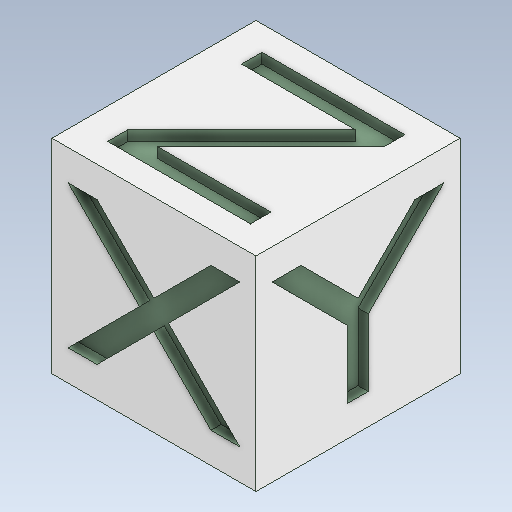
# Autodesk Inventor part: Cubo-0001-002
Saved by Autodesk Inventor 2025.2 (Build 292293000, 293)
## iProperties
Created: 2025-01-15
Part Number: Cubo-0001-002
Material: Borracha
Document SubType Name: Modeling
Designer: Gustavo Sousa
Density: 0.93 g/cm^3
Appearance: Borracha - Verde
Author: Gustavo Sousa
Autodesk Inventor part; units mm, degrees
ref_plane "YZ Plane" through (0, 0, 0) normal (1, 0, 0) x (0, 1, 0)
ref_plane "XZ Plane" through (0, 0, 0) normal (0, 1, 0) x (-1, 0, 0)
ref_plane "XY Plane" through (0, 0, 0) normal (0, 0, 1) x (1, 0, 0)
sketch "Esboço1" plane through (0, 0, 0) normal (0, 0, 1) x (1, 0, 0)
  line L0 (-10, -10) -> (10, -10)
  line L1 (10, -10) -> (10, 10)
  line L2 (10, 10) -> (-10, 10)
  line L3 (-10, 10) -> (-10, -10)
  line L4 (-10, -10) -> (10, 10) construction
  line L5 (10, -10) -> (-10, 10) construction
  point P0 (0, 0)
  dimension "d0" = 20
  dimension "d1" = 20
  constraints: 12 end point, 2 midpoint, 2 parallel, 1 horizontal, 1 perpendicular
  measures "d0" distance of L2.end L1.end
  measures "d1" distance of L1.end L0.end
extrude "Extrusão1" add sketch "Esboço1" along normal mid plane 20
sketch "Esboço4" plane through (0, 0, 10) normal (0, 0, 1) x (1, 0, 0)
  line L0 (-7, -7) -> (7, -7) construction
  line L1 (7, -7) -> (7, 7) construction
  line L2 (7, 7) -> (-7, 7) construction
  line L3 (-7, 7) -> (-7, -7) construction
  line L4 (0, 1.4142) -> (-1.4142, 0)
  line L5 (-1.4142, 0) -> (0, -1.4142)
  line L6 (0, -1.4142) -> (1.4142, 0)
  line L7 (1.4142, 0) -> (0, 1.4142)
  line L8 (0, 1.4142) -> (0, -1.4142) construction
  line L9 (-1.4142, 0) -> (1.4142, 0) construction
  line L10 (0, -1.4142) -> (1.4142, 0)
  line L11 (1.4142, 0) -> (7.0002, -5.586)
  line L12 (5.586, -7.0002) -> (0, -1.4142)
  line L13 (0, -1.4142) -> (-1.4142, 0)
  line L14 (-1.4142, 0) -> (-7.0001, -5.5859)
  line L15 (-5.5859, -7.0001) -> (0, -1.4142)
  line L16 (-1.4142, 0) -> (0, 1.4142)
  line L17 (0, 1.4142) -> (-5.5858, 7)
  line L18 (-7, 5.5858) -> (-1.4142, 0)
  line L19 (1.4142, 0) -> (0, 1.4142)
  line L20 (0, 1.4142) -> (5.5858, 7)
  line L21 (7, 5.5858) -> (1.4142, 0)
  line L22 (-8.4142, 7) -> (-7, 5.5858)
  line L23 (7, 5.5858) -> (8.4142, 7)
  line L24 (8.4142, -7) -> (7, -5.5858)
  line L25 (-7, -5.5858) -> (-8.4142, -7)
  line L26 (-5.5858, -7) -> (-8.4142, -7)
  line L27 (5.5858, -7) -> (7, -7)
  line L28 (7, -7) -> (8.4142, -7)
  line L29 (-5.5858, 7) -> (-8.4142, 7)
  line L30 (5.5858, 7) -> (7, 7)
  line L31 (7, 7) -> (8.4142, 7)
  point P0 (0, 0)
  point P1 (0, 0)
  point P2 (-7, 7)
  point P3 (-7, -7)
  point P4 (6.2929, 7)
  point P5 (7.7071, -7)
  dimension "d62" = 2
  dimension "d63" = 2
  dimension "d64" = 14
  dimension "d65" = 14
  dimension "d68" = 2
  dimension "d69" = 2
  dimension "d70" = 2
  dimension "d71" = 2
  constraints: 64 end point, 10 collinear, 8 parallel, 6 perpendicular, 4 horizontal, 4 midpoint, 1 vertical, 8 other
  measures "d62" distance of L6.end L5.end
  measures "d63" distance of L5.end L4.end
  measures "d64" distance of L2.end L0.start
  measures "d65" distance of L1.end L2.end
  measures "d68" distance of L29.start L22.end
  measures "d69" distance of L22.end L22.start
  measures "d70" distance of L23.end L23.start
  measures "d71" distance of L23.start L30.start
extrude "Extrusão4" cut sketch "Esboço4" against normal blind 1
sketch "Esboço7" plane through (10, -10, 10) normal (1, 0, 0) x (0, 0, -1)
  line L0 (17, 3) -> (3, 3) construction
  line L1 (3, 3) -> (3, 17) construction
  line L2 (3, 17) -> (17, 17) construction
  line L3 (17, 17) -> (17, 3) construction
  line L4 (8.5858, 10) -> (10, 11.4142) construction
  line L5 (10, 11.4142) -> (11.4142, 10) construction
  line L6 (11.4142, 10) -> (11, 9.5858) construction
  line L7 (9, 9.5858) -> (8.5858, 10) construction
  line L8 (8.5858, 10) -> (11.4142, 10) construction
  line L9 (10, 11.4142) -> (10, 8.5858) construction
  line L10 (10, 11.4142) -> (4.4142, 17)
  line L11 (3, 15.5858) -> (8.5858, 10)
  line L12 (10, 11.4142) -> (15.5858, 17)
  line L13 (17, 15.5858) -> (11.4142, 10)
  line L14 (18.4142, 17) -> (17, 15.5858) construction
  line L15 (15.5858, 17) -> (18.4142, 17) construction
  line L16 (3, 15.5858) -> (1.5858, 17) construction
  line L17 (1.5858, 17) -> (4.4142, 17) construction
  line L18 (4.4142, 17) -> (1.5858, 17)
  line L19 (3, 15.5858) -> (1.5858, 17)
  line L20 (15.5858, 17) -> (18.4142, 17)
  line L21 (17, 15.5858) -> (18.4142, 17)
  line L22 (8.5858, 10) -> (9, 9.5858)
  line L23 (11.4142, 10) -> (11, 9.5858)
  line L24 (9, 3) -> (11, 3)
  line L25 (11, 3) -> (11, 9.5858)
  line L26 (9, 9.5858) -> (9, 3)
  line L27 (8.5858, 10) -> (10, 8.5858) construction
  line L28 (10, 8.5858) -> (11.4142, 10) construction
  point P0 (10, 10)
  point P1 (4.4142, 17)
  point P2 (8.7929, 9.7929)
  constraints: 58 end point, 6 collinear, 6 parallel, 4 horizontal, 4 vertical, 3 point on line, 2 perpendicular, 1 midpoint, 8 other
extrude "Extrusão7" cut sketch "Esboço7" against normal blind 1
sketch "Esboço8" plane through (-10, 10, 10) normal (0, 1, 0) x (1, 0, 0)
  line L0 (17, 17.5858) -> (3, 17.5858) construction
  line L1 (10, 11.4142) -> (8.5858, 10) construction
  line L2 (8.5858, 10) -> (10, 8.5858) construction
  line L3 (10, 8.5858) -> (11.4142, 10) construction
  line L4 (11.4142, 10) -> (10, 11.4142) construction
  line L5 (10, 11.4142) -> (10, 8.5858) construction
  line L6 (8.5858, 10) -> (11.4142, 10) construction
  line L7 (11.4142, 10) -> (17, 15.5858)
  line L8 (14.1716, 15.5858) -> (10, 11.4142)
  line L9 (8.5858, 10) -> (3, 4.4142)
  line L10 (5.8712, 4.457) -> (10, 8.5858)
  line L11 (10, 11.4142) -> (8.5858, 10)
  line L12 (11.4142, 10) -> (10, 8.5858)
  line L13 (3, 4.4142) -> (3, 2.457)
  line L14 (17, 2.457) -> (17, 4.457)
  line L15 (17, 4.457) -> (5.8712, 4.457)
  line L16 (17, 17.5858) -> (17, 15.5858)
  line L17 (14.1716, 15.5858) -> (3, 15.5858)
  line L18 (3, 15.5858) -> (3, 17.5858)
  line L19 (3, 17.5858) -> (17, 17.5858)
  line L20 (3, 2.457) -> (17, 2.457)
  point P0 (10, 10)
  constraints: 42 end point, 6 parallel, 4 horizontal, 4 vertical, 3 perpendicular, 2 collinear, 3 other
extrude "Extrusão8" cut sketch "Esboço8" against normal blind 1
